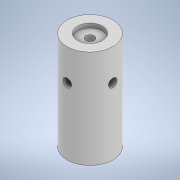
# Autodesk Inventor part: shaft
Saved by Autodesk Inventor 2020.3 (Build 243373000, 373)
## iProperties
Created: 2020-08-08
Part Number: shaft
Material: Generic
Document SubType Name: Modeling
Designer: joesp
Density: 1 g/cm^3
Appearance: Default
Author: joesp
Autodesk Inventor part; units mm, degrees
ref_plane "YZ Plane" through (0, 0, 0) normal (1, 0, 0) x (0, 1, 0)
ref_plane "XZ Plane" through (0, 0, 0) normal (0, 1, 0) x (-1, 0, 0)
ref_plane "XY Plane" through (0, 0, 0) normal (0, 0, 1) x (1, 0, 0)
sketch "Sketch1" plane through (0, 0, 0) normal (1, 0, 0) x (0, 1, 0)
  line L0 (0, 0) -> (45, 0)
  line L1 (45, 0) -> (45, -11)
  line L2 (45, -11) -> (0, -11)
  line L3 (0, -11) -> (0, 0)
  line L4 (0, -11) -> (45, -11)
  line L5 (45, -11) -> (45, -2)
  line L6 (45, -2) -> (0, -2)
  line L7 (0, -2) -> (0, -11)
  line L8 (45, -11) -> (47, -11)
  line L9 (47, -11) -> (47, -6)
  line L10 (47, -6) -> (45, -6)
  line L11 (45, -6) -> (45, -11)
  point P0 (0, -2)
  dimension "d1" = 11
  dimension "d2" = 45
  dimension "d39" = 2
  dimension "d40" = 2
  dimension "d41" = 5
  constraints: 24 end point, 6 parallel, 3 horizontal, 3 perpendicular, 1 coincident, 1 point on line
  measures "d1" distance of L0.end L1.end
  measures "d2" distance of L0.start L0.end
  measures "d39" distance between parallel lines of L0 L6
  measures "d40" distance of L4.end L8.end
  measures "d41" distance of L8.end L9.end
revolve "Revolution1" add sketch "Sketch1" angle 360 about axis through (0, 0, 0) along (0, 1, 0) contours L6 L1 L2 L3 | L10 L9 L8 L1
sketch "Sketch2" plane through (0, 0, 0) normal (1, 0, 0) x (0, 1, 0)
  circle A0 centre (32, 0) radius 2
  line L0 (45, 6) -> (45, -6) projected
  point P0 (0, 0)
  dimension "d8" = 4
  dimension "d42" = 13
  constraints: 1 centre point
  measures "d8" diameter of A0
  measures "d42" distance from line of L0 A0.centre
extrude "Extrusion1" cut sketch "Sketch2" along normal through all both and the other way through all
sketch "Sketch3" plane through (0, 0, 0) normal (0, 0, 1) x (1, 0, 0)
  circle A0 centre (0, 32) radius 2
  line L0 (-6, 45) -> (6, 45) projected
  point P0 (0, 0)
  dimension "d13" = 4
  dimension "d43" = 13
  constraints: 1 centre point, 1 vertical alignment
  measures "d13" diameter of A0
  measures "d43" distance from line of L0 A0.centre
extrude "Extrusion2" cut sketch "Sketch3" against normal through all both and the other way through all
body "Solid1"
